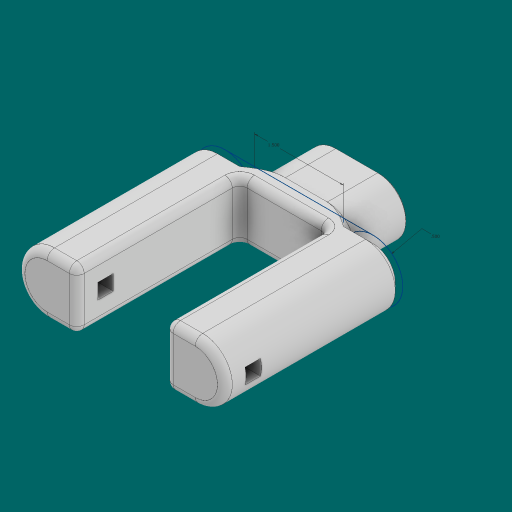
# Autodesk Inventor part: wheeltest
Saved by Autodesk Inventor 2023.1 (Build 271208000, 208)
## iProperties
Created: 2022-11-06
Part Number: wheeltest
Material: Generic
Document SubType Name: Modeling
Designer: zac-h
Density: 1 g/cm^3
Appearance: Default
Author: zac-h
## iProperties of the stored document wheeltest_3DPrint.ipt
Created: 2022-11-06
Part Number: wheeltest_3DPrint
Material: Generic
Document SubType Name: Modeling
Designer: zac-h
Density: 1 g/cm^3
Appearance: Default
Author: zac-h
Autodesk Inventor part; units mm, degrees
ref_plane "YZ Plane" through (0, 0, 0) normal (1, 0, 0) x (0, 1, 0)
ref_plane "XZ Plane" through (0, 0, 0) normal (0, 1, 0) x (-1, 0, 0)
ref_plane "XY Plane" through (0, 0, 0) normal (0, 0, 1) x (1, 0, 0)
sketch "Sketch1" plane through (0, 0, 0) normal (0, 0, 1) x (1, 0, 0)
  line L0 (-9, 0) -> (9, 0) construction
  line L1 (-9, -12) -> (9, -12)
  line L2 (9, 12) -> (-9, 12)
  arc A0 (-9, 12) -> (-9, -12) centre (-9, 0) ccw
  arc A1 (9, -12) -> (9, 12) centre (9, 0) ccw
  point P0 (0, 0)
  dimension "d11" = 12
  dimension "d12" = 18
  constraints: 8 end point, 4 point on circle, 4 tangent, 2 centre point, 1 horizontal, 1 midpoint, 1 parallel
  measures "d11" radius of A0
  measures "d12" distance of L2.start L2.end
extrude "Extrusion1" add sketch "Sketch1" along normal blind 25.4
sketch "Sketch2" plane through (0, 0, 25.4) normal (0, 0, 1) x (1, 0, 0)
  line L0 (-31.75, 0) -> (31.75, 0) construction
  line L1 (-31.75, -12.7) -> (31.75, -12.7)
  line L2 (31.75, 12.7) -> (-31.75, 12.7)
  arc A0 (-31.75, 12.7) -> (-31.75, -12.7) centre (-31.75, 0) ccw
  arc A1 (31.75, -12.7) -> (31.75, 12.7) centre (31.75, 0) ccw
  circle A2 centre (-31.75, 0) radius 12.7
  circle A3 centre (31.75, 0) radius 12.7
  line L3 (19.05, 0) -> (19.05, 12.7)
  line L4 (19.05, 0) -> (19.05, -12.7)
  line L5 (-19.05, 0) -> (-19.05, 12.7)
  line L6 (-19.05, 0) -> (-19.05, -12.7)
  point P0 (0, 0)
  dimension "d10" = 12.7
  dimension "d13" = 38.1
  constraints: 16 end point, 8 point on circle, 8 point on line, 6 tangent, 4 centre point, 2 coincident, 2 perpendicular, 1 horizontal, 1 midpoint, 1 parallel
  measures "d10" radius of A1
  measures "d13" distance between parallel lines of L3 L5
extrude "Extrusion2" add sketch "Sketch2" along normal blind 6.35
extrude "Extrusion3" add sketch "Sketch2" along normal blind 76.2 contours A2 L6 L1 | A0 A2 | L2 L5 A2 | L4 A3 L1 | A3 A1 | L3 L2 A3
sketch "Sketch3" plane through (-19.05, -12.7, 31.75) normal (1, 0, 0) x (0, 0, -1)
  line L0 (-60.7776, 9.398) -> (-54.1736, 9.398)
  line L1 (-54.1736, 9.398) -> (-54.1736, 16.002)
  line L2 (-54.1736, 16.002) -> (-60.7776, 16.002)
  line L3 (-60.7776, 16.002) -> (-60.7776, 9.398)
  line L4 (-60.7776, 9.398) -> (-54.1736, 16.002) construction
  line L5 (-54.1736, 9.398) -> (-60.7776, 16.002) construction
  point P0 (31.75, 12.7)
  point P1 (-57.4756, 12.7)
  dimension "d6" = 6.604
  dimension "d7" = 6.604
  constraints: 12 end point, 2 midpoint, 2 parallel, 1 horizontal, 1 perpendicular
  measures "d6" distance of L2.end L1.end
  measures "d7" distance of L1.end L0.end
extrude "Extrusion4" cut sketch "Sketch3" along normal through all both and the other way through all
fillet "Fillet1" radius 3.175 2 edges at (-19.05, 0, 31.75) (19.05, 0, 31.75)
fillet "Fillet2" radius 3.175 2 edges at (-19.05, 0, 101.6) (19.05, 0, 101.6)
fillet "Fillet3" radius 3.175 20 edges at (-19.9799, 12.7, 100.6701) (-26.9875, 12.7, 101.6) (-44.45, 0, 101.6) (-26.9875, -12.7, 101.6) (-19.9799, -12.7, 100.6701) (-19.05, -12.7, 66.675) (-18.1201, -12.7, 32.6799) (0, -12.7, 31.75) (18.1201, -12.7, 32.6799) (19.05, -12.7, 66.675) (19.9799, -12.7, 100.6701) (26.9875, -12.7, 101.6) (44.45, 0, 101.6) (26.9875, 12.7, 101.6) (19.9799, 12.7, 100.6701) (19.05, 12.7, 66.675) (18.1201, 12.7, 32.6799) (0, 12.7, 31.75) (-18.1201, 12.7, 32.6799) (-19.05, 12.7, 66.675)
chamfer "Chamfer1" distance 3.175 angle 45 4 edges at (21, 0, 25.4) (0, 12, 25.4) (-21, 0, 25.4) (0, -12, 25.4)
chamfer "Chamfer2" distance 3.175 angle 45 6 edges at (-44.45, 0, 25.4) (-24.528, -12.7, 25.4) (-24.528, 12.7, 25.4) (44.45, 0, 25.4) (24.528, 12.7, 25.4) (24.528, -12.7, 25.4)
chamfer "Chamfer3" distance 0.6 angle 45 4 edges at (0, 12, 0) (-21, 0, 0) (0, -12, 0) (21, 0, 0)
body "Solid1"
